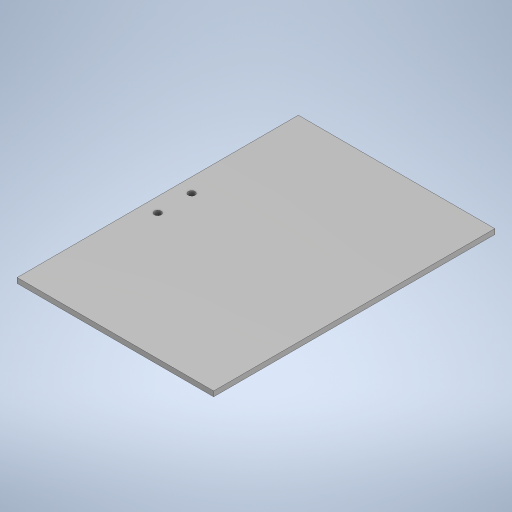
# Autodesk Inventor part: pcb
Saved by Autodesk Inventor 2024 (Build 280153000, 153)
## iProperties
Created: 2024-03-09
Part Number: pcb
Material: PBT Plastic
Document SubType Name: Modeling
Designer: kdcao
Density: 1.31 g/cm^3
Appearance: Smooth - Medium Gray
Author: kdcao
Autodesk Inventor part; units mm, degrees
ref_plane "YZ Plane" through (0, 0, 0) normal (1, 0, 0) x (0, 1, 0)
ref_plane "XZ Plane" through (0, 0, 0) normal (0, 1, 0) x (-1, 0, 0)
ref_plane "XY Plane" through (0, 0, 0) normal (0, 0, 1) x (1, 0, 0)
sketch "Sketch1" plane through (0, 0, 0) normal (0, 1, 0) x (-1, 0, 0)
  line L0 (-29, 41.5) -> (29, 41.5)
  line L1 (29, 41.5) -> (29, -41.5)
  line L2 (29, -41.5) -> (-29, -41.5)
  line L3 (-29, -41.5) -> (-29, 41.5)
  line L4 (-29, 41.5) -> (29, -41.5) construction
  line L5 (29, 41.5) -> (-29, -41.5) construction
  point P0 (0, 0)
  dimension "d0" = 83
  dimension "d1" = 58
  constraints: 12 end point, 2 midpoint, 2 parallel, 1 horizontal, 1 perpendicular
  measures "d0" distance of L0.end L1.end
  measures "d1" distance of L0.start L0.end
extrude "Extrusion1" add sketch "Sketch1" along normal blind 1.5
sketch "Sketch2" plane through (0, 1.5, 0) normal (0, 1, 0) x (1, 0, 0)
  line L0 (-29, 41.5) -> (-29, -41.5) projected
  point P0 (0, 0)
  point P1 (-24.75, 5.75)
  point P2 (-24.75, -4.25)
  point P3 (-29, 0)
  dimension "d11" = 10
  dimension "d12" = 4.25
  dimension "d13" = 4.25
  dimension "d14" = 5.75
  constraints: 1 midpoint
  measures "d11" distance of point (-24.75, 5.75) point (-24.75, -4.25)
  measures "d12" distance from line of L0 point (-24.75, -4.25)
  measures "d13" distance from line of L0 point (-24.75, 5.75)
  measures "d14" vertical distance of point (-29, 0) point (-24.75, 5.75)
hole "Hole1" at (-24.75, 1.5, -5.75) at (-24.75, 1.5, 4.25) direction (0, -1, 0) diameter 2 end through all
body "Solid1"
